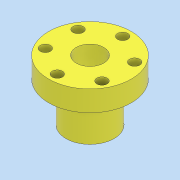
# Autodesk Inventor part: Nakrętka trapezowa kołnierzowa JFRM-2835TR16x4
Saved by Autodesk Inventor 2018 (Build 220112000, 112)
## iProperties
Created: 2019-01-25
Part Number: Nakrętka trapezowa kołnierzowa JFRM-2835TR16x4
Material: Ogólny
Document SubType Name: Modeling
Designer: Dawid
Density: 1 g/cm^3
Appearance: Domyślna
Author: Dawid
Autodesk Inventor part; units mm, degrees
ref_plane "YZ Plane" through (0, 0, 0) normal (1, 0, 0) x (0, 1, 0)
ref_plane "XZ Plane" through (0, 0, 0) normal (0, 1, 0) x (-1, 0, 0)
ref_plane "XY Plane" through (0, 0, 0) normal (0, 0, 1) x (1, 0, 0)
sketch "Szkic1" plane through (0, 0, 0) normal (0, 0, 1) x (1, 0, 0)
  circle A0 centre (0, 0) radius 24
  circle A1 centre (0, 0) radius 8
  dimension "d0" = 48
  dimension "d1" = 16
  constraints: 2 centre point, 2 coincident
  measures "d0" diameter of A0
  measures "d1" diameter of A1
extrude "Wyciągnięcie proste1" add sketch "Szkic1" along normal blind 12
sketch "Szkic2" plane through (0, 0, 0) normal (0, 0, -1) x (-1, 0, 0)
  circle A0 centre (0, 0) radius 8 projected
  circle A1 centre (0, 0) radius 14
  dimension "d4" = 28
  constraints: 1 centre point, 1 coincident
  measures "d4" diameter of A1
extrude "Wyciągnięcie proste2" add sketch "Szkic2" along normal blind 23
sketch "Szkic3" plane through (0, 0, 12) normal (0, 0, 1) x (1, 0, 0)
  circle A0 centre (0, 0) radius 19
  circle A1 centre (0, 19) radius 3
  circle A2 centre (16.4545, 9.5) radius 3
  circle A3 centre (16.4545, -9.5) radius 3
  circle A4 centre (0, -19) radius 3
  circle A5 centre (-16.4545, -9.5) radius 3
  circle A6 centre (-16.4545, 9.5) radius 3
  dimension "d7" = 38
  dimension "d8" = 6
  dimension "d11" = 360
  constraints: 6 centre point, 1 coincident, 1 vertical alignment, 15 other
  measures "d8" diameter of A1
extrude "Wyciągnięcie proste3" cut sketch "Szkic3" against normal up to next contours A2 A0 | A0 A2 | A3 A0 | A0 A3 | A1 A0 | A0 A1 | A4 A0 | A0 A4 | A6 A0 | A0 A6 | A5 A0 | A0 A5
